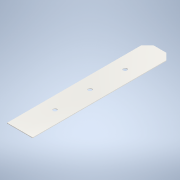
# Autodesk Inventor part: Horquilla_Base
Saved by Autodesk Inventor 2022.1 (Build 261234000, 234)
## iProperties
Created: 2021-09-10
Part Number: Horquilla_Base
Material: Genérico
Document SubType Name: Modeling
Designer: seb_0
Density: 1 g/cm^3
Appearance: Acero
Author: seb_0
Autodesk Inventor part; units mm, degrees
ref_plane "YZ Plane" through (0, 0, 0) normal (1, 0, 0) x (0, 1, 0)
ref_plane "XZ Plane" through (0, 0, 0) normal (0, 1, 0) x (-1, 0, 0)
ref_plane "XY Plane" through (0, 0, 0) normal (0, 0, 1) x (1, 0, 0)
sketch "Boceto1" plane through (0, 0, 0) normal (0, 1, 0) x (-1, 0, 0)
  line L0 (0, 0) -> (200, 0)
  line L1 (200, 0) -> (200, -1050)
  line L2 (150, -1100) -> (50, -1100)
  line L3 (0, -1050) -> (0, 0)
  line L4 (200, -1050) -> (150, -1100)
  line L5 (0, -1050) -> (50, -1100)
  circle A0 centre (100, -550) radius 15
  circle A1 centre (100, -825) radius 15
  circle A2 centre (100, -275) radius 15
  point P0 (200, -1100)
  point P1 (0, -1100)
  point P2 (100, 0)
  dimension "d0" = 1100
  dimension "d1" = 200
  dimension "d2" = 50
  dimension "d3" = 50
  dimension "d4" = 50
  dimension "d5" = 50
  dimension "d6" = 30
  dimension "d7" = 100
  dimension "d12" = 30
  dimension "d13" = 30
  dimension "d14" = 100
  dimension "d15" = 275
  dimension "d16" = 275
  dimension "d17" = 275
  dimension "d18" = 100
  constraints: 12 end point, 4 point on line, 3 centre point, 2 parallel, 1 horizontal, 1 midpoint, 1 perpendicular
  measures "d0" distance of L0.end point (200, -1100)
  measures "d1" distance of point (200, -1100) point (0, -1100)
  measures "d2" distance of L1.end point (200, -1100)
  measures "d3" distance of L2.start point (200, -1100)
  measures "d4" distance of L3.start point (0, -1100)
  measures "d5" distance of L2.end point (0, -1100)
  measures "d6" diameter of A0
  measures "d7" distance from line of L3 A0.centre
  measures "d12" diameter of A1
  measures "d13" diameter of A2
  measures "d14" distance from line of L3 A2.centre
  measures "d15" distance from line of L0 A2.centre
  measures "d16" distance of A0.centre A2.centre
  measures "d17" distance of A1.centre A0.centre
  measures "d18" distance from line of L3 A1.centre
extrude "Extrusión1" add sketch "Boceto1" along normal blind 3
equation "\"d3\" = d2"
equation "\"d4\" = d2"
equation "\"d5\" = d4"
